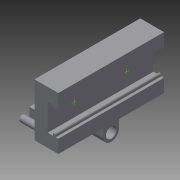
# Autodesk Inventor part: Karetka
Saved by Autodesk Inventor 2015 (Build 190159000, 159)
## iProperties
Created: 2016-04-08
Part Number: Karetka
Material: Generic
Document SubType Name: Modeling
Designer: Andreas
Density: 1 g/cm^3
Appearance: Default
Author: Andreas
Autodesk Inventor part; units mm, degrees
ref_plane "YZ Plane" through (0, 0, 0) normal (1, 0, 0) x (0, 1, 0)
ref_plane "XZ Plane" through (0, 0, 0) normal (0, 1, 0) x (-1, 0, 0)
ref_plane "XY Plane" through (0, 0, 0) normal (0, 0, 1) x (1, 0, 0)
sketch "Sketch1" plane through (0, 0, 0) normal (0, 1, 0) x (-1, 0, 0)
  line L0 (0, 0) -> (0, 5)
  line L1 (0, 5) -> (9, 5)
  line L2 (9, 5) -> (9, -15)
  line L3 (9, -15) -> (0, -15)
  line L4 (0, -15) -> (0, -10)
  line L5 (0, -10) -> (4, -10)
  line L6 (4, -10) -> (4, 0)
  line L7 (4, 0) -> (0, 0)
  dimension "d0" = 5
  dimension "d1" = 9
  dimension "d2" = 20
  dimension "d3" = 9
  dimension "d4" = 5
  dimension "d5" = 4
  dimension "d6" = 10
  constraints: 16 end point, 5 perpendicular, 2 vertical
  measures "d0" distance of L0.start L0.end
  measures "d1" distance of L0.end L1.end
  measures "d2" distance of L1.end L2.end
  measures "d3" distance of L2.end L3.end
  measures "d4" distance of L3.end L4.end
  measures "d5" distance of L4.end L5.end
  measures "d6" distance of L5.end L6.end
extrude "Extrusion1" add sketch "Sketch1" along normal blind 40
sketch "Sketch5" plane through (0, 0, 0) normal (0, -1, 0) x (1, 0, 0)
  line L0 (-1, -10) -> (-1, -9.5)
  line L1 (-1.5, -9) -> (-1.5, -9)
  line L2 (-2, -9.5) -> (-2, -10)
  line L3 (-2, -10) -> (-1, -10)
  line L4 (-1, -0.5) -> (-1, 0)
  line L5 (-1, 0) -> (-2, 0)
  line L6 (-2, 0) -> (-2, -0.5)
  line L7 (-1.5, -1) -> (-1.5, -1)
  arc A0 (-1.5, -9) -> (-2, -9.5) centre (-1.5, -9.5) ccw
  arc A1 (-1, -9.5) -> (-1.5, -9) centre (-1.5, -9.5) ccw
  arc A2 (-2, -0.5) -> (-1.5, -1) centre (-1.5, -0.5) ccw
  arc A3 (-1.5, -1) -> (-1, -0.5) centre (-1.5, -0.5) ccw
  point P0 (0, 0)
  point P1 (-1, -9)
  point P2 (-2, -9)
  point P3 (-1, -1)
  point P4 (-2, -1)
  point P5 (-1.5, 0)
  point P6 (-1.5, -10)
  point P7 (0, -10)
  dimension "d35" = 1
  dimension "d36" = 1
  dimension "d37" = 1
  dimension "d38" = 1
  dimension "d39" = 1
  dimension "d40" = 1
  dimension "d41" = 0.5
  dimension "d42" = 1
  dimension "d43" = 1
  constraints: 16 end point, 10 point on line, 8 point on circle, 8 tangent, 4 centre point, 3 equal radius, 3 perpendicular, 2 horizontal alignment, 2 midpoint, 1 horizontal, 1 vertical
  measures "d35" distance of L0.start point (-1, -9)
  measures "d36" distance of point (-1, -9) point (-2, -9)
  measures "d37" distance of point (-2, -9) L2.end
  measures "d38" distance of point (-1, -1) L4.end
  measures "d39" distance of L4.end L5.end
  measures "d40" distance of L5.end point (-2, -1)
  measures "d41" radius of A0
  measures "d42" distance from line of point (0, -10) L0
  measures "d43" horizontal distance of point (0, 0) L4.start
extrude "Extrusion2" add sketch "Sketch5" against normal blind 40
sketch "Sketch7" plane through (-9, 0, -15) normal (-1, 0, 0) x (0, 0, 1)
  line L0 (5, 0) -> (5, 5)
  line L1 (5, 0) -> (5, 40) projected
  line L2 (5, 5) -> (0, 5)
  line L3 (0, 0) -> (0, 40) projected
  line L4 (0, 35) -> (5, 35)
  line L5 (5, 40) -> (5, 0)
  line L6 (0, 0) -> (5, 0) projected
  circle A0 centre (2.5, 2.5) radius 1.25
  circle A1 centre (2.5, 37.5) radius 1.25
  point P0 (15, 0)
  dimension "d51" = 5
  dimension "d52" = 2.5
  dimension "d53" = 2.5
  constraints: 8 end point, 4 point on line, 2 centre point, 2 perpendicular, 1 parallel
  measures "d51" distance of L0.start L0.end
  measures "d52" diameter of A0
  measures "d53" diameter of A1
extrude "Extrusion4" add sketch "Sketch7" along normal blind 7 contours L2 L3 L4 L1 | A0 | A1
sketch "Sketch8" plane through (-16, 0, -15) normal (-1, 0, 0) x (0, 0, 1)
  line L0 (0, 40) -> (20, 40) projected
  line L1 (20, 0) -> (0, 0) projected
  line L2 (0, 40) -> (0, 23)
  line L3 (0, 0) -> (0, 40) projected
  line L4 (0, 23) -> (-3, 23)
  line L5 (0, 0) -> (0, 17)
  line L6 (0, 17) -> (-3, 17)
  arc A0 (-3, 23) -> (-3, 17) centre (-3, 20) ccw
  circle A1 centre (-3, 20) radius 2
  point P0 (15, 0)
  dimension "d56" = 40
  dimension "d57" = 17
  dimension "d58" = 3
  dimension "d59" = 17
  dimension "d60" = 3
  dimension "d61" = 4
  constraints: 8 end point, 2 centre point, 2 perpendicular, 2 point on circle, 2 point on line, 1 coincident, 1 tangent
  measures "d56" distance between parallel lines of L0 L1
  measures "d57" distance of L0.start L2.end
  measures "d58" distance of L2.end L4.end
  measures "d59" distance of L1.end L5.end
  measures "d60" distance of L5.end L6.end
  measures "d61" diameter of A1
extrude "Extrusion5" add sketch "Sketch8" against normal blind 16
sketch "Sketch4" plane through (-4, 0, 0) normal (1, 0, 0) x (0, 0, -1)
  point P0 (5, 30)
  point P1 (5, 10)
body "Solid1"
